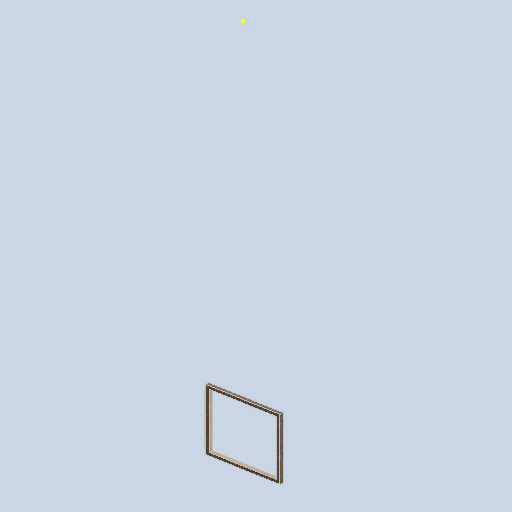
# Autodesk Inventor part: eave_frame_side
Saved by Autodesk Inventor 2024.2 (Build 282272000, 272)
## iProperties
Created: 2024-05-23
Part Number: eave_frame_side
Material: Wood (Maple)
Document SubType Name: Modeling
Designer: LOSTER_1
Density: 0.67 g/cm^3
Appearance: Natural Maple - Glossy Dark Tint
Author: LOSTER_1
Autodesk Inventor part; units mm, degrees
ref_plane "XZ Plane" through (0, 0, 0) normal (0, 1, 0) x (-1, 0, 0)
ref_plane "XY Plane" through (0, 0, 0) normal (0, 0, 1) x (1, 0, 0)
sketch "Sketch1" plane through (0, 0, 0) normal (1, 0, 0) x (0, 1, 0)
  line L0 (-11549.3083, -1493.8295) -> (-11549.3083, 1506.1705)
  line L1 (-13549.3083, -1493.8295) -> (-13549.3083, 1506.1705)
  line L2 (-13724.3083, 1506.1705) -> (-13724.3083, -1493.8295)
  line L3 (-13724.3083, 1506.1705) -> (-11374.3083, 1506.1705)
  line L4 (-11374.3083, 1506.1705) -> (-11374.3083, -1493.8295)
  line L5 (-13724.3083, 1506.1705) -> (-11374.3083, 1506.1705)
  line L6 (-11374.3083, 1506.1705) -> (-11374.3083, 1356.1705)
  line L7 (-11374.3083, 1356.1705) -> (-13724.3083, 1356.1705)
  line L8 (-13724.3083, 1356.1705) -> (-13724.3083, 1506.1705)
  point P0 (0, 0)
  point P1 (-13549.3083, 1506.1705)
  dimension "d2" = 150
  constraints: 18 end point, 2 coincident, 2 horizontal, 2 parallel, 2 perpendicular, 1 point on line, 1 vertical
  measures "d2" distance of L5.end L6.end
ref_plane "Work Plane2" through (2500, 0, 0) normal (1, 0, 0) x (0, 1, 0)
ref_plane "Work Plane1" through (0, 0, 0) normal (1, 0, 0) x (0, 1, 0)
extrude "Extrusion1" add sketch "Sketch1" along normal blind 60
sketch "Sketch2" plane through (60, 0, 0) normal (1, 0, 0) x (0, 0, -1)
  point P0 (0, 0)
ref_plane "Work Plane3" through (60, 0, 0) normal (1, 0, 0) x (0, 0, -1)
sketch "Sketch3" plane through (2500, 0, 0) normal (1, 0, 0) x (0, 1, 0)
  line L0 (-11374.3083, 1506.1705) -> (-11374.3083, -1493.8295) projected
  line L1 (-13724.3083, 1506.1705) -> (-13724.3083, -1493.8295) projected
  point P0 (0, 0)
ref_plane "Work Plane4" through (0, -13724.3083, 1506.1705) normal (0, -1, 0) x (0, 0, -1)
sketch "Sketch4" plane through (0, -13724.3083, 1506.1705) normal (0, -1, 0) x (0, 0, -1)
  line L0 (0, 60) -> (150, 60) projected
  line L1 (0, 2500) -> (3000, 2500) projected
  line L2 (0, 60) -> (430.2378, 2500)
  line L3 (0, 60) -> (2477.6409, 60) construction
  line L4 (150, 60) -> (580.2378, 2500)
  line L5 (150, 60) -> (2627.6409, 60) construction
  line L6 (580.2378, 2500) -> (430.2378, 2500)
  line L7 (0, 60) -> (150, 60)
  point P0 (1506.1705, 0)
  dimension "d6" = 80
  dimension "d7" = 80
  constraints: 12 end point, 2 collinear, 2 equal length, 2 horizontal, 2 point on line
  measures "d6" angle of L3 L2
  measures "d7" angle of L5 L4
sketch "Sketch5" plane through (2500, 0, 0) normal (1, 0, 0) x (0, 1, 0)
  line L0 (-13724.3083, 1506.1705) -> (-13724.3083, -1493.8295) projected
  line L1 (-11374.3083, 1506.1705) -> (-11374.3083, -1493.8295) projected
  line L2 (-13724.3083, 1075.9326) -> (-11374.3083, 1075.9326)
  line L3 (-11374.3083, 1075.9326) -> (-11374.3083, 925.9326)
  line L4 (-11374.3083, 925.9326) -> (-13724.3083, 925.9326)
  line L5 (-13724.3083, 925.9326) -> (-13724.3083, 1075.9326)
  point P0 (0, 0)
  constraints: 8 end point, 2 parallel, 1 horizontal, 1 perpendicular, 1 point on line
loft "Loft1" add profiles "Sketch5" section 2 edges at (60, -11374.3083, 1431.1705) (60, -12549.3083, 1506.1705) (60, -13724.3083, 1431.1705) (60, -12549.3083, 1356.1705)
sketch "Sketch6" plane through (0, -13724.3083, 1506.1705) normal (0, 0, 1) x (1, 0, 0)
  line L0 (60, 2350) -> (60, 0) projected
  line L1 (0, 2175) -> (60, 2175)
  line L2 (60, 2175) -> (60, 2350)
  line L3 (60, 2350) -> (0, 2350)
  line L4 (0, 2350) -> (0, 2175)
  line L5 (0, 175) -> (60, 175)
  line L6 (60, 175) -> (60, 0)
  line L7 (60, 0) -> (0, 0)
  line L8 (0, 0) -> (0, 175)
  point P0 (0, 13724.3083)
  constraints: 16 end point, 4 parallel, 2 horizontal, 2 perpendicular
extrude "Extrusion2" cut sketch "Sketch6" against normal through all
sketch "Sketch7" plane through (0, -13724.3083, 1506.1705) normal (0, -1, 0) x (0, 0, -1)
  line L0 (0, 60) -> (150, 60) projected
  line L1 (150, 60) -> (575.438, 2472.779)
  line L2 (150, 0) -> (150, 60) projected
  line L3 (150, 60) -> (120, 60)
  line L4 (120, 60) -> (545.438, 2472.779)
  line L5 (545.438, 2472.779) -> (575.438, 2472.779)
  line L6 (430.2378, 2500) -> (580.2378, 2500) projected
  point P0 (1506.1705, 0)
  dimension "d15" = 2450
  dimension "d16" = 30
  dimension "d17" = 2450
  constraints: 8 end point, 2 coincident, 1 parallel, 1 point on line
  measures "d15" distance of L0.end L1.end
  measures "d16" distance of L0.end L3.end
  measures "d17" distance of L3.end L4.end
extrude "Extrusion3" cut sketch "Sketch7" against normal through all
sketch "Sketch8" plane through (0, 0, 0) normal (-1, 0, 0) x (0, 0, 1)
  point P0 (0, 0)
sketch "Sketch9" plane through (0, -13549.3083, 1506.1705) normal (0, 0, 1) x (1, 0, 0)
  line L0 (2500, -175) -> (2500, 2175) projected
  line L1 (2500, 2175) -> (60, 2175) projected
  line L2 (60, 2175) -> (60, 2000) projected
  line L3 (60, 2000) -> (60, 0) projected
  line L4 (60, 0) -> (60, -175) projected
  line L5 (2500, -175) -> (60, -175) projected
  line L6 (60, -175) -> (180, -175)
  line L7 (180, -175) -> (180, -55)
  line L8 (180, -55) -> (60, -55)
  line L9 (60, -55) -> (60, -175)
  line L10 (2500, 2175) -> (2380, 2175)
  line L11 (2380, 2175) -> (2380, 2055)
  line L12 (2380, 2055) -> (2500, 2055)
  line L13 (2500, 2055) -> (2500, 2175)
  line L14 (2380, 2055) -> (180, 2055)
  line L15 (180, 2055) -> (180, -55)
  line L16 (180, -55) -> (2380, -55)
  line L17 (2380, -55) -> (2380, 2055)
  point P0 (0, 13549.3083)
  dimension "d20" = 120
  dimension "d21" = 120
  dimension "d22" = 120
  dimension "d23" = 120
  constraints: 24 end point, 6 parallel, 3 horizontal, 3 perpendicular
  measures "d20" distance of L8.end L7.end
  measures "d21" distance of L7.end L6.end
  measures "d22" distance of L12.end L11.end
  measures "d23" distance of L11.end L10.end
extrude "Extrusion4" cut sketch "Sketch9" against normal through all contours L17 L16 L15 L14
body "Solid1"
